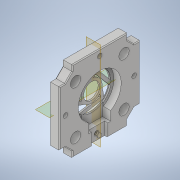
# Autodesk Inventor part: 20_Cube_Insert_VCA_base_lower_v0
Saved by Autodesk Inventor 2022.3 (Build 263350000, 350)
## iProperties
Created: 2019-07-01
Part Number: 20_Cube_Insert_VCA_base_lower_v0
Material: Generic
Document SubType Name: Modeling
Designer: diederichbenedict
Density: 1 g/cm^3
Appearance: Default
Author: diederichbenedict
Autodesk Inventor part; units mm, degrees
ref_plane "YZ Plane" through (0, 0, 0) normal (1, 0, 0) x (0, 1, 0)
ref_plane "XZ Plane" through (0, 0, 0) normal (0, 1, 0) x (-1, 0, 0)
ref_plane "Work Plane1" through (3.0022, -38.4528, -56.3184) normal (-1, 0, 0) x (0, -1, 0)
sketch "Sketch1" plane through (3.0022, -38.4528, -56.3184) normal (-1, 0, 0) x (0, -1, 0)
  line L0 (-4.0299, -0.3538) -> (-2.2322, 1.4439) construction
  arc A0 (-1.4439, 2.2322) -> (-2.2322, 1.4439) centre (-0.9299, 0.9299) ccw construction
  line L1 (-1.4439, 2.2322) -> (0.3538, 4.0299) construction
  line L2 (-37.8299, 42.8299) -> (-37.8299, 37.8299) construction
  line L3 (-37.8299, 37.8299) -> (-42.9208, 37.8299) construction
  line L4 (-37.8299, 42.2137) -> (-37.8299, 45.8299) construction
  line L5 (-37.8299, 45.8299) -> (-4.0299, 45.8299) construction
  line L6 (-4.0299, 45.8299) -> (-4.0299, 42.2137) construction
  line L7 (-4.0299, 4.0299) -> (0.3538, 4.0299) projected
  circle A1 centre (-20.9299, 20.9299) radius 17.5 projected
  line L8 (-20.9299, 58.9723) -> (17.1124, 20.9299) construction
  line L9 (17.1124, 20.9299) -> (-20.9299, -17.1124) construction
  line L10 (-20.9299, -17.1124) -> (-58.9723, 20.9299) construction
  line L11 (-58.9723, 20.9299) -> (-20.9299, 58.9723) construction
  line L12 (-20.9299, 58.9723) -> (-20.9299, -17.1124) construction
  line L13 (17.1124, 20.9299) -> (-58.9723, 20.9299) construction
  line L14 (-20.9299, 58.9723) -> (32.8701, 58.9723) construction
  line L15 (-43.4299, 43.4299) -> (1.5701, 43.4299) construction
  line L16 (1.5701, 43.4299) -> (1.5701, -1.5701) construction
  line L17 (1.5701, -1.5701) -> (-43.4299, -1.5701) construction
  line L18 (-43.4299, -1.5701) -> (-43.4299, 43.4299) construction
  line L19 (-43.4299, 43.4299) -> (1.5701, -1.5701) construction
  line L20 (1.5701, 43.4299) -> (-43.4299, -1.5701) construction
  line L21 (-43.4299, 5.3876) -> (-43.4299, 36.4723)
  line L22 (-43.4299, 36.4723) -> (-36.4723, 43.4299)
  line L23 (-36.4723, 43.4299) -> (-5.3876, 43.4299)
  line L24 (-5.3876, 43.4299) -> (1.5701, 36.4723)
  line L25 (1.5701, 36.4723) -> (1.5701, 5.3876)
  line L26 (1.5701, 5.3876) -> (-5.3876, -1.5701)
  line L27 (-5.3876, -1.5701) -> (-36.4723, -1.5701)
  line L28 (-36.4723, -1.5701) -> (-43.4299, 5.3876)
  line L29 (-4.0299, 42.2137) -> (-37.8299, 42.2137) projected
  line L30 (-4.0299, -0.3538) -> (-4.0299, 4.0299) projected
  circle A2 centre (-20.9299, 20.9299) radius 1.5
  line L31 (-10.9299, 10.9299) -> (-30.9299, 10.9299) construction
  line L32 (-30.9299, 10.9299) -> (-30.9299, 30.9299) construction
  line L33 (-30.9299, 30.9299) -> (-10.9299, 30.9299) construction
  line L34 (-10.9299, 30.9299) -> (-10.9299, 10.9299) construction
  line L35 (-10.9299, 10.9299) -> (-30.9299, 30.9299) construction
  line L36 (-30.9299, 10.9299) -> (-10.9299, 30.9299) construction
  circle A3 centre (-30.9299, 30.9299) radius 1.4
  circle A4 centre (-30.9299, 10.9299) radius 1.4
  circle A5 centre (-10.9299, 10.9299) radius 1.4
  line L37 (-45.8299, 37.8299) -> (-42.0723, 37.8299) construction
  line L38 (-42.1723, 37.7299) -> (-45.8299, 37.7299)
  line L39 (-45.8299, 37.7299) -> (-45.8299, 4.1299)
  line L40 (-45.8299, 4.1299) -> (-42.1723, 4.1299)
  line L41 (-42.1723, 4.1299) -> (-42.1723, 37.7299)
  line L42 (-45.8299, 4.0299) -> (-42.0723, 4.0299) construction
  line L43 (-45.8299, 37.8299) -> (-42.0723, 37.8299) projected
  line L44 (-37.7299, 45.8299) -> (-4.1299, 45.8299)
  line L45 (-4.1299, 45.8299) -> (-4.1299, 42.1723)
  line L46 (-4.1299, 42.1723) -> (-37.7299, 42.1723)
  line L47 (-37.7299, 42.1723) -> (-37.7299, 45.8299)
  line L48 (0.4701, 37.8299) -> (0.4701, 4.0299) construction
  line L49 (0.4701, 4.0299) -> (3.9701, 4.0299) construction
  line L50 (3.9701, 37.8299) -> (3.9701, 4.0299) construction
  line L51 (0.4701, 37.8299) -> (3.9701, 37.8299) construction
  line L52 (-45.8299, -3.9701) -> (-4.0299, -3.9701) construction
  line L53 (0.3124, 37.7299) -> (3.9701, 37.7299)
  line L54 (3.9701, 37.7299) -> (3.9701, 4.1299)
  line L55 (3.9701, 4.1299) -> (0.3124, 4.1299)
  line L56 (0.3124, 4.1299) -> (0.3124, 37.7299)
  line L57 (-4.1713, -0.3538) -> (-37.7299, -0.3538)
  line L58 (-37.7299, -0.3538) -> (-37.7299, -3.9701)
  line L59 (-37.7299, -3.9701) -> (-4.1713, -3.9701)
  line L60 (-4.1713, -3.9701) -> (-4.1713, -0.3538)
  point P0 (-37.8299, 4.0299)
  dimension "d18" = 53.8
  dimension "d19" = 45
  dimension "d20" = 53.8
  dimension "d21" = 45
  dimension "d22" = 45
  dimension "d30" = 20
  dimension "d31" = 20
  dimension "d32" = 2.8
  dimension "d33" = 2.8
  dimension "d34" = 2.8
  dimension "d35" = 3
  dimension "d36" = 0.1
  dimension "d37" = 0.1
  dimension "d38" = 0.1
  dimension "d39" = 0.1
  constraints: 86 end point, 21 point on line, 14 parallel, 8 perpendicular, 7 horizontal, 7 midpoint, 4 centre point, 4 coincident, 1 equal length
  measures "d18" distance of L8.start L8.end
  measures "d19" angle of L8 L14
  measures "d20" distance of L8.end L9.end
  measures "d21" distance of L16.end L17.end
  measures "d22" distance of L15.end L16.end
  measures "d30" distance of L32.end L33.end
  measures "d31" distance of L31.end L32.end
  measures "d32" diameter of A3
  measures "d33" diameter of A4
  measures "d34" diameter of A5
  measures "d35" diameter of A2
  measures "d36" distance between parallel lines of L38 L43
  measures "d37" distance between parallel lines of L40 L42
  measures "d38" distance between parallel lines of L45 L6
  measures "d39" distance between parallel lines of L4 L47
extrude "Extrusion1" add sketch "Sketch1" along normal blind 6 contours L30 L26 L57 L28 L41 L22 L46 L24 L56 L7 | L7 L26 L30 | L56 L24 L25 L26 | L26 L25 L24 L53 L54 L55 | L60 L59 L58 L57 L28 L27 L26 | L26 L27 L28 L57 | L46 L22 L29 L24 | L24 L29 L45 | L40 L39 L38 L22 L21 L28 | L28 L21 L22 L41 | L29 L22 L23 L24 | L24 L23 L22 L29 L47 L44 L45 | L47 L29 L22 | A1 | A2 | A3 | A4 | A5
sketch "Skizze4" plane through (-2.9978, -38.4528, -56.3184) normal (-1, 0, 0) x (0, -1, 0)
  line L0 (-37.7299, 42.1723) -> (-42.1723, 37.7299) projected
  line L1 (-42.1723, 37.7299) -> (-45.8299, 37.7299) projected
  line L2 (-45.8299, 37.7299) -> (-45.8299, 4.1299) construction
  line L3 (-45.8299, 4.1299) -> (-42.1723, 4.1299) projected
  line L4 (-42.1723, 4.1299) -> (-37.6885, -0.3538) projected
  line L5 (-37.6885, -0.3538) -> (-37.7299, -0.3538) projected
  line L6 (-37.7299, -0.3538) -> (-37.7299, -3.9701) projected
  line L7 (-37.7299, -3.9701) -> (-4.1713, -3.9701) construction
  line L8 (-4.1713, -3.9701) -> (-4.1713, -0.3538) projected
  line L9 (-4.1713, -0.3538) -> (0.3124, 4.1299) projected
  line L10 (0.3124, 4.1299) -> (3.9701, 4.1299) projected
  line L11 (3.9701, 4.1299) -> (3.9701, 37.7299) construction
  line L12 (3.9701, 37.7299) -> (0.3124, 37.7299) projected
  line L13 (0.3124, 37.7299) -> (-4.1299, 42.1723) projected
  line L14 (-4.1299, 42.1723) -> (-4.1299, 45.8299) projected
  line L15 (-4.1299, 45.8299) -> (-37.7299, 45.8299) construction
  line L16 (-37.7299, 45.8299) -> (-37.7299, 42.1723) projected
  line L17 (-37.9299, 46.0299) -> (-3.9299, 46.0299) construction
  line L18 (-3.9299, 46.0299) -> (-3.9299, 42.2551)
  line L19 (-3.9299, 42.2551) -> (0.3953, 37.9299)
  line L20 (0.3953, 37.9299) -> (4.1701, 37.9299)
  line L21 (4.1701, 37.9299) -> (4.1701, 3.9299) construction
  line L22 (4.1701, 3.9299) -> (0.3953, 3.9299)
  line L23 (0.3953, 3.9299) -> (-3.9713, -0.4367)
  line L24 (-3.9713, -0.4367) -> (-3.9713, -4.1701)
  line L25 (-3.9713, -4.1701) -> (-37.9299, -4.1701) construction
  line L26 (-37.9299, -4.1701) -> (-37.9299, -0.3953)
  line L27 (-37.9299, -0.3953) -> (-42.2551, 3.9299)
  line L28 (-42.2551, 3.9299) -> (-46.0299, 3.9299)
  line L29 (-46.0299, 3.9299) -> (-46.0299, 37.9299) construction
  line L30 (-46.0299, 37.9299) -> (-42.2551, 37.9299)
  line L31 (-42.2551, 37.9299) -> (-37.9299, 42.2551)
  line L32 (-37.9299, 42.2551) -> (-37.9299, 46.0299)
  line L33 (-45.8299, 37.7299) -> (-45.8299, 37.9299)
  line L34 (-4.1299, 45.8299) -> (-37.7299, 45.8299) projected
  line L35 (-37.7299, 45.8299) -> (-37.9299, 45.8299)
  line L36 (-4.1299, 45.8299) -> (-3.9299, 45.8299)
  line L37 (3.9701, 37.7299) -> (3.9701, 37.9299)
  line L38 (3.9701, 4.1299) -> (3.9701, 37.7299) projected
  line L39 (3.9701, 4.1299) -> (3.9701, 3.9299)
  line L40 (-4.1713, -3.9701) -> (-3.9713, -3.9701)
  line L41 (-37.7299, -3.9701) -> (-37.9299, -3.9701)
  line L42 (-45.8299, 4.1299) -> (-45.8299, 3.9299)
  point P0 (-38.4528, 56.3184)
  dimension "d40" = 0.2
  constraints: 48 end point, 12 point on line, 4 perpendicular, 15 other
  measures "d40" distance between parallel lines of L15 L17
extrude "IM_offset" add sketch "Skizze4" against normal up to surface (6 mm away)
ref_plane "Arbeitsebene5" through (3.0022, -17.5229, -52.3885) normal (0, -1, 0) x (1, 0, 0)
ref_plane "Arbeitsebene6" through (3.0022, -0.5229, -35.3885) normal (0, 0, 1) x (0, -1, 0)
sketch "Skizze31" plane through (-2.9978, -38.4528, -56.3184) normal (-1, 0, 0) x (0, -1, 0)
  line L0 (3.9701, 3.9299) -> (3.9701, 37.9299) projected
  line L1 (3.9701, 37.9299) -> (0.3953, 37.9299) projected
  line L2 (0.3953, 37.9299) -> (-3.9299, 42.2551) projected
  line L3 (-3.9299, 42.2551) -> (-3.9299, 45.8299) projected
  line L4 (-3.9299, 45.8299) -> (-37.9299, 45.8299) projected
  line L5 (-37.9299, 45.8299) -> (-37.9299, 42.2551) projected
  line L6 (-37.9299, 42.2551) -> (-42.2551, 37.9299) projected
  line L7 (-42.2551, 37.9299) -> (-45.8299, 37.9299) projected
  line L8 (-45.8299, 37.9299) -> (-45.8299, 3.9299) projected
  line L9 (-42.2551, 3.9299) -> (-45.8299, 3.9299) projected
  line L10 (-37.9299, -0.3953) -> (-42.2551, 3.9299) projected
  line L11 (-37.9299, -3.9701) -> (-37.9299, -0.3953) projected
  line L12 (-3.9713, -3.9701) -> (-37.9299, -3.9701) projected
  line L13 (-3.9713, -3.9701) -> (-3.9713, -0.4367) projected
  line L14 (-3.9713, -0.4367) -> (0.3953, 3.9299) projected
  line L15 (0.3953, 3.9299) -> (3.9701, 3.9299) projected
  circle A0 centre (-20.9506, 20.9092) radius 11.5
  arc A1 (-17.516, 31.8843) -> (-32.4478, 21.1639) centre (-20.9506, 20.9092) ccw projected
  point P0 (-38.4528, 56.3184)
  dimension "d181" = 23
  constraints: 1 centre point
  measures "d181" diameter of A0
extrude "Extrusion26" cut sketch "Skizze31" against normal blind 10 contours A0
chamfer "Fase2" distance 0.5 angle 45 34 edges at (3.0022, -17.5229, -10.4885) (3.0022, -0.5229, -12.2759) (3.0022, 1.6397, -16.2259) (3.0022, 5.5897, -18.3885) (3.0022, 7.3771, -35.3885) (3.0022, 5.5897, -52.3885) (3.0022, 1.6397, -54.5511) (3.0022, -0.5229, -58.5011) (3.0022, -17.5022, -60.2885) (3.0022, -34.4815, -58.5218) (3.0022, -36.6648, -54.5718) (3.0022, -40.6355, -52.3885) (3.0022, -42.4229, -35.3885) (3.0022, -40.6355, -18.3885) (3.0022, -36.6855, -16.2259) (-2.9978, -36.6648, -54.5718) (-2.9978, -40.6355, -52.3885) (-2.9978, -42.4229, -35.3885) (-2.9978, -34.4815, -58.5218) (-2.9978, -17.5022, -60.2885) (-2.9978, -0.5229, -58.5011) (-2.9978, 1.6397, -54.5511) (-2.9978, 5.5897, -52.3885) (-2.9978, 7.3771, -35.3885) (-2.9978, 5.5897, -18.3885) (-2.9978, 1.6397, -16.2259) (-2.9978, -0.5229, -12.2759) (-2.9978, -17.5229, -10.4885) (-2.9978, -34.5229, -12.2759) (-2.9978, -36.6855, -16.2259) (-2.9978, -40.6355, -18.3885) (-2.9978, -6.0022, -35.4092) (3.0022, -6.0022, -35.4092) (3.0022, -34.5229, -12.2759)
sketch "Skizze32" plane through (3.0022, -38.4528, -56.3184) normal (1, 0, 0) x (0, 1, 0)
  line L0 (4.8056, 6.489) -> (64.0062, 6.489) construction
  line L1 (64.0062, 6.489) -> (64.0062, -0.9654) construction
  line L2 (64.0062, -0.9654) -> (4.8056, -0.9654) construction
  line L3 (4.8056, -0.9654) -> (4.8056, 6.489) construction
  point P0 (38.4528, 56.3184)
  constraints: 2 other
extrude "Extrusion27" [suppressed]
sketch "Skizze33" plane through (3.0022, -38.4528, -56.3184) normal (1, 0, 0) x (0, 1, 0)
  circle A0 centre (20.9506, 20.9092) radius 13 construction
  circle A1 centre (20.9506, 20.9092) radius 13.25
  point P0 (38.4528, 56.3184)
  dimension "d189" = 26.5
  constraints: 1 centre point, 1 coincident
  measures "d189" diameter of A1
extrude "Extrusion28" cut sketch "Skizze33" against normal blind 4.5
sketch "Skizze34" plane through (3.0022, -38.4528, -56.3184) normal (1, 0, 0) x (0, 1, 0)
  arc A0 (13.1444, 27.1592) -> (13.1444, 14.6592) centre (20.9506, 20.9092) ccw projected
  line L0 (13.1444, 27.1592) -> (6.3506, 27.1592) projected
  line L1 (6.3506, 27.1592) -> (6.3506, 14.6592) projected
  line L2 (6.3506, 14.6592) -> (13.1444, 14.6592) projected
  arc A1 (14.2658, 27.6592) -> (14.2658, 14.1592) centre (20.9506, 20.9092) ccw
  line L3 (14.2658, 27.6592) -> (5.8506, 27.6592)
  line L4 (5.8506, 27.6592) -> (5.8506, 14.1592)
  line L5 (5.8506, 14.1592) -> (14.2658, 14.1592)
  line L6 (5.8506, 27.6592) -> (3.8506, 27.6592)
  line L7 (3.8506, 27.6592) -> (3.8506, 14.1592)
  line L8 (3.8506, 14.1592) -> (5.8506, 14.1592)
  line L9 (5.8506, 14.1592) -> (5.8506, 27.6592)
  point P0 (38.4528, 56.3184)
  point P1 (5.8506, 14.1592)
  dimension "d192" = 0.5
  dimension "d225" = 2
  constraints: 14 end point, 2 parallel, 2 point on circle, 1 centre point, 1 horizontal, 1 perpendicular, 3 other
  measures "d192" distance between parallel lines of L2 L5
  measures "d225" distance of L8.end L7.end
extrude "Extrusion29" cut sketch "Skizze34" against normal through all contours A0 L2 L1 L0 | A1 L5 L4 L3 | L4 L8 L7 L6
sketch "Skizze35" plane through (-2.9978, -38.4528, -56.3184) normal (-1, 0, 0) x (0, -1, 0)
  circle A0 centre (-20.9092, 20.9092) radius 11.5
  circle A1 centre (-20.9092, 20.9092) radius 12.0343
  line L0 (-3.8506, 14.1592) -> (-11.0291, 14.1592) projected
  line L1 (-3.8506, 27.6592) -> (-3.8506, 14.1592) projected
  line L2 (-11.0291, 27.6592) -> (-3.8506, 27.6592) projected
  arc A2 (-14.0321, 59.1067) -> (-14.0321, 53.5302) centre (-17.2396, 56.3184) ccw projected
  line L3 (-14.0321, 39.8391) -> (-14.0321, 53.5302) projected
  line L4 (-17.314, 39.8391) -> (-14.0321, 39.8391) projected
  line L5 (-21.9321, 35.2211) -> (-17.314, 39.8391) projected
  line L6 (-21.9321, 31.9391) -> (-21.9321, 35.2211) projected
  line L7 (-35.6176, 31.9391) -> (-21.9321, 31.9391) projected
  arc A3 (-35.6176, 31.9391) -> (-41.288, 31.9391) centre (-38.4528, 35.1052) ccw projected
  line L8 (-54.9321, 31.9391) -> (-41.288, 31.9391) projected
  line L9 (-54.9321, 35.2211) -> (-54.9321, 31.9391) projected
  line L10 (-59.5502, 39.8391) -> (-54.9321, 35.2211) projected
  line L11 (-62.8321, 39.8391) -> (-59.5502, 39.8391) projected
  line L12 (-62.8321, 53.4832) -> (-62.8321, 39.8391) projected
  arc A4 (-62.8321, 53.4832) -> (-62.8321, 59.1536) centre (-59.666, 56.3184) ccw projected
  line L13 (-62.8321, 72.7977) -> (-62.8321, 59.1536) projected
  line L14 (-59.5916, 72.7977) -> (-62.8321, 72.7977) projected
  line L15 (-54.9321, 77.4572) -> (-59.5916, 72.7977) projected
  line L16 (-54.9321, 80.7391) -> (-54.9321, 77.4572) projected
  line L17 (-41.2411, 80.7391) -> (-54.9321, 80.7391) projected
  arc A5 (-41.2411, 80.7391) -> (-35.6646, 80.7391) centre (-38.4528, 77.5316) ccw projected
  line L18 (-21.9321, 80.7391) -> (-35.6646, 80.7391) projected
  line L19 (-21.9321, 77.4572) -> (-21.9321, 80.7391) projected
  line L20 (-17.314, 72.8391) -> (-21.9321, 77.4572) projected
  line L21 (-14.0321, 72.8391) -> (-17.314, 72.8391) projected
  line L22 (-14.0321, 59.1067) -> (-14.0321, 72.8391) projected
  circle A6 centre (-53.4528, 71.277) radius 4.1599 projected
  circle A7 centre (-23.4528, 71.277) radius 4.1599 projected
  line L23 (-45.2028, 71.4184) -> (-45.2028, 65.7175) projected
  line L24 (-28.6289, 62.2896) -> (-28.6233, 62.2876) projected
  arc A8 (-28.6233, 62.2876) -> (-29.0707, 62.9686) centre (-38.4528, 56.3184) ccw projected
  line L25 (-31.7028, 65.6515) -> (-31.7028, 71.4184) projected
  line L26 (-31.7028, 71.4184) -> (-45.2028, 71.4184) projected
  line L27 (-40.9659, 45.0964) -> (-40.9613, 45.1003) projected
  arc A9 (-41.9828, 45.3736) -> (-40.9659, 45.0964) centre (-38.4528, 56.3184) ccw projected
  line L28 (-27.4777, 59.7531) -> (-27.4961, 59.7596) projected
  line L29 (-38.178, 44.8384) -> (-38.1981, 44.8213) projected
  arc A10 (-38.1981, 44.8213) -> (-27.4777, 59.7531) centre (-38.4528, 56.3184) ccw projected
  circle A11 centre (-53.4528, 41.3599) radius 4.1599 projected
  circle A12 centre (-23.4528, 41.3599) radius 4.1599 projected
  arc A13 (-29.0707, 62.9686) -> (-31.7028, 65.6515) centre (-38.4984, 56.3519) ccw projected
  arc A14 (-45.2028, 65.7175) -> (-41.9828, 45.3736) centre (-38.4984, 56.3519) ccw projected
  arc A15 (-40.9613, 45.1003) -> (-38.178, 44.8384) centre (-38.4984, 56.3519) ccw projected
  arc A16 (-27.4961, 59.7596) -> (-28.6289, 62.2896) centre (-38.4984, 56.3519) ccw projected
  point P0 (-38.4528, 56.3184)
  point P1 (-13.1218, 29.3712)
  point P2 (-11.5986, 27.6592)
  point P3 (-14.9401, 11.0797)
  point P4 (-11.5986, 14.1592)
  point P5 (-32.1313, 23.4223)
  point P6 (-15.3812, 30.9934)
  point P7 (-10.9462, 27.6592)
  point P8 (-10.9462, 14.1592)
  constraints: 1 centre point, 1 coincident, 7 other
extrude "Extrusion30" add sketch "Skizze35" against normal blind 1 contours A0 L6 A1 L7 | A0 L7 A1 L6 | L2 L1 L0 A1
sketch "Skizze37" plane through (-1.9978, -38.4528, -56.3184) normal (1, 0, 0) x (0, 1, 0)
  line L0 (28.6233, 62.2876) -> (28.6249, 62.283) projected
  line L1 (16.1488, 13.6368) -> (14.2659, 12.9626) projected
  arc A0 (14.0321, 53.5302) -> (14.0321, 59.1067) centre (17.2396, 56.3184) ccw projected
  line L2 (14.0321, 39.8391) -> (14.0321, 53.5302) projected
  line L3 (17.314, 39.8391) -> (14.0321, 39.8391) projected
  line L4 (21.9321, 35.2211) -> (17.314, 39.8391) projected
  line L5 (21.9321, 31.9391) -> (21.9321, 35.2211) projected
  line L6 (35.6176, 31.9391) -> (21.9321, 31.9391) projected
  arc A1 (41.288, 31.9391) -> (35.6176, 31.9391) centre (38.4528, 35.1052) ccw projected
  line L7 (54.9321, 31.9391) -> (41.288, 31.9391) projected
  line L8 (54.9321, 35.2211) -> (54.9321, 31.9391) projected
  line L9 (59.5502, 39.8391) -> (54.9321, 35.2211) projected
  line L10 (62.8321, 39.8391) -> (59.5502, 39.8391) projected
  line L11 (62.8321, 53.4832) -> (62.8321, 39.8391) projected
  arc A2 (62.8321, 59.1536) -> (62.8321, 53.4832) centre (59.666, 56.3184) ccw projected
  line L12 (62.8321, 72.7977) -> (62.8321, 59.1536) projected
  line L13 (59.5916, 72.7977) -> (62.8321, 72.7977) projected
  line L14 (54.9321, 77.4572) -> (59.5916, 72.7977) projected
  line L15 (54.9321, 80.7391) -> (54.9321, 77.4572) projected
  line L16 (41.2411, 80.7391) -> (54.9321, 80.7391) projected
  arc A3 (35.6646, 80.7391) -> (41.2411, 80.7391) centre (38.4528, 77.5316) ccw projected
  line L17 (21.9321, 80.7391) -> (35.6646, 80.7391) projected
  line L18 (21.9321, 77.4572) -> (21.9321, 80.7391) projected
  line L19 (17.314, 72.8391) -> (21.9321, 77.4572) projected
  line L20 (14.0321, 72.8391) -> (17.314, 72.8391) projected
  line L21 (14.0321, 59.1067) -> (14.0321, 72.8391) projected
  circle A4 centre (53.4528, 71.277) radius 4.1599 projected
  circle A5 centre (23.4528, 71.277) radius 4.1599 projected
  line L22 (45.2028, 71.4184) -> (45.2028, 65.7175) projected
  line L23 (28.6289, 62.2896) -> (28.6233, 62.2876) projected
  arc A6 (29.0707, 62.9686) -> (28.6233, 62.2876) centre (38.4528, 56.3184) ccw projected
  line L24 (31.7028, 65.6515) -> (31.7028, 71.4184) projected
  line L25 (31.7028, 71.4184) -> (45.2028, 71.4184) projected
  line L26 (40.9659, 45.0964) -> (40.9613, 45.1003) projected
  arc A7 (40.9659, 45.0964) -> (41.9828, 45.3736) centre (38.4528, 56.3184) ccw projected
  line L27 (27.4777, 59.7531) -> (27.4961, 59.7596) projected
  line L28 (38.178, 44.8384) -> (38.1981, 44.8213) projected
  arc A8 (27.4777, 59.7531) -> (38.1981, 44.8213) centre (38.4528, 56.3184) ccw projected
  circle A9 centre (53.4528, 41.3599) radius 4.1599 projected
  circle A10 centre (23.4528, 41.3599) radius 4.1599 projected
  line L29 (12.9546, 22.558) -> (11.0717, 21.8838) projected
  line L30 (11.7458, 20.0008) -> (13.6288, 20.675) projected
  line L31 (26.3144, 26.9737) -> (26.672, 28.9415) projected
  line L32 (24.7042, 29.2991) -> (24.3466, 27.3314) projected
  line L33 (16.9913, 28.668) -> (17.349, 30.6358) projected
  line L34 (15.3812, 30.9934) -> (15.0236, 29.0256) projected
  line L35 (38.1981, 44.8213) -> (38.2119, 44.8375) projected
  line L36 (29.5875, 20.4228) -> (31.1128, 19.1292) projected
  line L37 (26.2776, 13.4277) -> (24.7523, 14.7213) projected
  line L38 (23.4587, 13.1959) -> (24.984, 11.9024) projected
  arc A11 (31.7028, 65.6515) -> (29.0707, 62.9686) centre (38.4984, 56.3519) ccw projected
  arc A12 (41.9828, 45.3736) -> (45.2028, 65.7175) centre (38.4984, 56.3519) ccw projected
  arc A13 (38.178, 44.8384) -> (40.9613, 45.1003) centre (38.4984, 56.3519) ccw projected
  arc A14 (28.6289, 62.2896) -> (27.4961, 59.7596) centre (38.4984, 56.3519) ccw projected
  point P0 (38.4528, 56.3184)
  point P1 (32.1313, 23.4223)
  point P2 (26.2779, 16.5203)
  point P3 (30.6806, 26.9731)
  point P4 (24.5043, 12.3092)
  point P5 (25.3181, 14.2414)
  point P6 (30.6806, 26.9731)
  constraints: 4 other
extrude "Extrusion31" cut sketch "Skizze37" against normal blind 0.5 contours L28 A13 L35
sketch "Skizze38" plane through (-2.9978, -38.4528, -56.3184) normal (-1, 0, 0) x (0, -1, 0)
  circle A0 centre (-35.9092, 5.9092) radius 3.1599
  circle A1 centre (-35.9092, 35.9092) radius 3.1599
  arc A2 (-32.1727, 18.3961) -> (-15.4226, 10.825) centre (-20.9506, 20.9092) ccw projected
  circle A3 centre (-5.9921, 35.9092) radius 3.1599
  circle A4 centre (-5.9921, 5.9092) radius 3.1599
  point P0 (-38.4528, 56.3184)
  point P1 (-9.7286, 23.4223)
  dimension "d207" = 180
  constraints: 4 centre point, 10 other
extrude "Extrusion32" cut sketch "Skizze38" against normal through all
sketch "Skizze39" plane through (-2.9978, -38.4528, -56.3184) normal (-1, 0, 0) x (0, -1, 0)
  line L0 (-4.4713, -3.4701) -> (-37.4299, -3.4701) projected
  line L1 (-4.4713, -0.2296) -> (-4.4713, -3.4701) projected
  line L2 (0.1882, 4.4299) -> (-4.4713, -0.2296) projected
  line L3 (3.4701, 4.4299) -> (0.1882, 4.4299) projected
  line L4 (3.4701, 37.4299) -> (3.4701, 4.4299) projected
  line L5 (0.1882, 37.4299) -> (3.4701, 37.4299) projected
  line L6 (-4.4299, 42.048) -> (0.1882, 37.4299) projected
  line L7 (-4.4299, 45.3299) -> (-4.4299, 42.048) projected
  line L8 (-37.4299, 45.3299) -> (-4.4299, 45.3299) projected
  line L9 (-37.4299, 42.048) -> (-37.4299, 45.3299) projected
  line L10 (-42.048, 37.4299) -> (-37.4299, 42.048) projected
  line L11 (-45.3299, 37.4299) -> (-42.048, 37.4299) projected
  line L12 (-45.3299, 4.4299) -> (-45.3299, 37.4299) projected
  line L13 (-42.048, 4.4299) -> (-45.3299, 4.4299) projected
  line L14 (-37.4299, -0.1882) -> (-42.048, 4.4299) projected
  line L15 (-37.4299, -3.4701) -> (-37.4299, -0.1882) projected
  line L16 (-20.9506, -0.304) -> (0.2626, 20.9092) construction
  line L17 (0.2626, 20.9092) -> (-20.9506, 42.1224) construction
  line L18 (-20.9506, 42.1224) -> (-42.1638, 20.9092) construction
  line L19 (-42.1638, 20.9092) -> (-20.9506, -0.304) construction
  line L20 (-20.9506, -0.304) -> (-20.9506, 42.1224) construction
  line L21 (0.2626, 20.9092) -> (-42.1638, 20.9092) construction
  line L22 (-20.9506, -0.304) -> (9.0494, -0.304) construction
  arc A0 (-30.8722, 27.6592) -> (-30.8722, 14.1592) centre (-20.9506, 20.9092) ccw projected
  arc A1 (-30.8722, 27.6592) -> (-30.8722, 14.1592) centre (-20.9092, 20.9092) ccw projected
  point P0 (-38.4528, 56.3184)
  dimension "d209" = 30
  dimension "d210" = 45
  dimension "d211" = 30
  constraints: 14 end point, 2 parallel, 1 equal length, 1 horizontal, 1 perpendicular
  measures "d209" distance of L16.start L16.end
  measures "d210" angle of L22 L16
  measures "d211" distance of L17.end L16.end
hole "Bohrung2" at (-2.9978, -17.5022, -56.6224) at (-2.9978, 3.711, -35.4092) at (-2.9978, -17.5022, -14.196) at (-2.9978, -38.7154, -35.4092) direction (1, 0, 0) diameter 2.8 end through all counterbore diameter 6.5 counterbore depth 3
sketch "Skizze40" plane through (3.0022, -38.4528, -56.3184) normal (1, 0, 0) x (0, 1, 0)
  circle A0 centre (-0.304, 20.9092) radius 1.4
  line L0 (-6.3758, 15.9092) -> (5.8506, 15.9092)
  line L1 (5.8506, 15.9092) -> (5.8506, 25.9092)
  line L2 (5.8506, 25.9092) -> (-6.3758, 25.9092)
  line L3 (-6.3758, 25.9092) -> (-6.3758, 15.9092)
  circle A1 centre (-0.2626, 20.9092) radius 1.4 projected
  line L4 (-6.3758, 15.9092) -> (5.8506, 25.9092) construction
  line L5 (5.8506, 15.9092) -> (-6.3758, 25.9092) construction
  point P0 (38.4528, 56.3184)
  point P1 (-0.2833, 19.5094)
  point P2 (-0.2833, 22.3091)
  dimension "d219" = 10
  constraints: 12 end point, 2 midpoint, 2 parallel, 1 centre point, 1 perpendicular, 2 other
  measures "d219" distance of L1.end L0.end
extrude "Extrusion33" cut sketch "Skizze40" against normal blind 2 contours A0 A1 | L3 L2 L1 L0 picked at (-0.7364, 20.9092)
chamfer "Fase4" distance 1 angle 45 11 edges at (-2.9978, -29.3008, -20.4092) (-2.9978, -40.8201, -32.9328) (-2.9978, -36.239, -37.514) (-2.9978, -29.3008, -50.4092) (-2.9978, -20.7311, -56.2532) (-2.9978, -14.2732, -56.2532) (-2.9978, 0.6163, -50.4092) (-2.9978, 1.1667, -37.4313) (-2.9978, 5.7331, -32.8649) (-2.9978, 0.6163, -20.4092) (-2.9978, -17.5022, -17.446)
sketch "Sketch41" plane through (-2.9978, -38.4528, -56.3184) normal (-1, 0, 0) x (0, 0, 1)
  arc A0 (30.2198, 27.6592) -> (26.8784, 30.7387) centre (20.9092, 20.9092) ccw
  arc A1 (28.6966, 12.4472) -> (30.2198, 14.1592) centre (20.9092, 20.9092) ccw
  line L0 (28.6966, 12.4472) -> (15.5041, 14.8447)
  line L1 (15.5041, 14.8447) -> (15.8619, 16.8136)
  arc A2 (15.8619, 16.8136) -> (24.7442, 15.6611) centre (20.9092, 20.9092) ccw
  line L2 (24.7442, 15.6611) -> (31.421, 18.0517)
  line L3 (31.421, 18.0517) -> (26.8784, 30.7387)
  arc A3 (19.886, 27.3282) -> (14.4467, 20.2121) centre (20.9092, 20.9092) ccw
  line L4 (14.4467, 20.2121) -> (13.1787, 13.2345)
  line L5 (13.1787, 13.2345) -> (26.4372, 10.825)
  arc A4 (9.6872, 18.3961) -> (26.4372, 10.825) centre (20.9092, 20.9092) ccw
  line L6 (9.6872, 18.3961) -> (18.3598, 28.6225)
  line L7 (18.3598, 28.6225) -> (19.886, 27.3282)
  circle A5 centre (20.9092, 20.9092) radius 5
  circle A6 centre (29.1592, 35.1986) radius 1.4
  circle A7 centre (4.4092, 20.9092) radius 1.4
  circle A8 centre (29.1592, 6.6198) radius 1.4
  line L8 (24.3438, 31.8843) -> (28.8638, 19.2605)
  line L9 (28.8638, 19.2605) -> (26.9798, 18.5859)
  arc A9 (26.9798, 18.5859) -> (23.5367, 26.8545) centre (20.9092, 20.9092) ccw
  line L10 (23.5367, 26.8545) -> (18.128, 31.4414)
  line L11 (18.128, 31.4414) -> (9.412, 21.1639)
  arc A10 (24.3438, 31.8843) -> (9.412, 21.1639) centre (20.9092, 20.9092) ccw
  circle A11 centre (20.9092, 20.9092) radius 19.3
  arc A12 (45.3299, 23.7389) -> (45.3299, 18.1624) centre (42.1224, 20.9506) ccw projected
  line L12 (45.3299, 37.4299) -> (45.3299, 23.7389) projected
  line L13 (42.048, 37.4299) -> (45.3299, 37.4299) projected
  line L14 (37.4299, 42.048) -> (42.048, 37.4299) projected
  line L15 (37.4299, 45.3299) -> (37.4299, 42.048) projected
  line L16 (23.7444, 45.3299) -> (37.4299, 45.3299) projected
  arc A13 (18.074, 45.3299) -> (23.7444, 45.3299) centre (20.9092, 42.1638) ccw projected
  line L17 (4.4299, 45.3299) -> (18.074, 45.3299) projected
  line L18 (4.4299, 42.048) -> (4.4299, 45.3299) projected
  line L19 (-0.1882, 37.4299) -> (4.4299, 42.048) projected
  line L20 (-3.4701, 37.4299) -> (-0.1882, 37.4299) projected
  line L21 (-3.4701, 23.7858) -> (-3.4701, 37.4299) projected
  arc A14 (-3.4701, 18.1154) -> (-3.4701, 23.7858) centre (-0.304, 20.9506) ccw projected
  line L22 (-3.4701, 4.4713) -> (-3.4701, 18.1154) projected
  line L23 (-0.2296, 4.4713) -> (-3.4701, 4.4713) projected
  line L24 (4.4299, -0.1882) -> (-0.2296, 4.4713) projected
  line L25 (4.4299, -3.4701) -> (4.4299, -0.1882) projected
  line L26 (18.121, -3.4701) -> (4.4299, -3.4701) projected
  arc A15 (23.6975, -3.4701) -> (18.121, -3.4701) centre (20.9092, -0.2626) ccw projected
  line L27 (37.4299, -3.4701) -> (23.6975, -3.4701) projected
  line L28 (37.4299, -0.1882) -> (37.4299, -3.4701) projected
  line L29 (42.048, 4.4299) -> (37.4299, -0.1882) projected
  line L30 (45.3299, 4.4299) -> (42.048, 4.4299) projected
  line L31 (45.3299, 18.1624) -> (45.3299, 4.4299) projected
  circle A16 centre (5.9092, 5.9921) radius 4.1599 projected
  circle A17 centre (35.9092, 5.9921) radius 4.1599 projected
  circle A18 centre (20.9092, 20.9092) radius 11.5 projected
  arc A19 (27.6592, 30.8722) -> (14.1592, 30.8722) centre (20.9092, 20.9506) ccw projected
  arc A20 (27.6592, 30.8722) -> (14.1592, 30.8722) centre (20.9092, 20.9092) ccw projected
  circle A21 centre (5.9092, 35.9092) radius 4.1599 projected
  circle A22 centre (35.9092, 35.9092) radius 4.1599 projected
  arc A23 (30.2198, 14.1592) -> (30.5295, 14.6084) centre (20.9092, 20.9092) ccw
  arc A24 (32.4029, 20.5276) -> (30.2198, 27.6592) centre (20.9092, 20.9092) ccw
  arc A25 (30.5295, 14.6084) -> (32.4029, 20.5276) centre (20.9092, 20.9092) ccw
  point P0 (56.3184, 38.4528)
  point P1 (-56.3599, 0)
  point P2 (9.6872, 18.3961)
  point P3 (26.4372, 10.825)
  point P4 (28.6966, 12.4472)
  point P5 (26.8784, 30.7387)
  point P6 (24.3438, 31.8843)
  constraints: 24 end point, 20 point on circle, 15 centre point, 2 point on line
extrude "Extrusion34" add sketch "Sketch41" against normal blind 1 contours L3 L2 A2 L1 L0 A18 L5 L4 A3 L7 L6 L11 L10 A9 L9 L8
body "Solid1"
